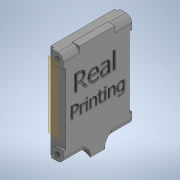
# Autodesk Inventor part: Partcooling_Brace
Saved by Autodesk Inventor 2022 (Build 260153000, 153)
## iProperties
Created: 2021-11-28
Part Number: Partcooling_Brace
Material: Polycarbonate, Clear
Document SubType Name: Modeling
Designer: alexr
Density: 1.2 g/cm^3
Appearance: Polycarbonate - Clear
Mass: 4.68895 g
Surface Area: 35.8129 cm^2
Volume: 3.90746 cm^3
Author: alexr
Autodesk Inventor part; units mm, degrees
ref_plane "YZ Plane" through (0, 0, 0) normal (1, 0, 0) x (0, 1, 0)
ref_plane "XZ Plane" through (0, 0, 0) normal (0, 1, 0) x (-1, 0, 0)
ref_plane "XY Plane" through (0, 0, 0) normal (0, 0, 1) x (1, 0, 0)
sketch "Sketch1" plane through (0, 0, 0) normal (1, 0, 0) x (0, 1, 0)
  line L0 (-12.75, -13.5) -> (12.75, -13.5)
  line L1 (12.75, -13.5) -> (12.75, 13.5)
  line L2 (12.75, 13.5) -> (-12.75, 13.5)
  line L3 (-12.75, 13.5) -> (-12.75, -13.5)
  line L4 (-12.75, -13.5) -> (12.75, 13.5) construction
  line L5 (12.75, -13.5) -> (-12.75, 13.5) construction
  dimension "d0" = 25.5
  dimension "d1" = 27
  constraints: 12 end point, 2 parallel, 1 horizontal, 1 perpendicular
  measures "d0" distance of L2.end L1.end
  measures "d1" distance of L1.end L0.end
extrude "Extrusion1" add sketch "Sketch1" along normal blind 6.25
ref_plane "Work Plane1" through (0, -12.75, 14.5) normal (0, 0, 1) x (1, 0, 0)
sketch "Sketch2" plane through (0, -12.75, 14.5) normal (0, 0, 1) x (1, 0, 0)
  arc A0 (6.25, 27.5) -> (3.75, 30) centre (3.75, 27.5) ccw projected
  line L0 (6.25, 27.5) -> (6.25, 25) projected
  line L1 (3.7511, 25) -> (6.25, 25) projected
  arc A1 (1.25, 27.5011) -> (3.7511, 25) centre (3.75, 27.5) ccw projected
  line L2 (1.25, 30) -> (1.25, 27.5011) projected
  line L3 (1.25, 30) -> (3.75, 30) projected
  circle A2 centre (3.75, 27.5) radius 1 projected
  arc A3 (3.75, -10) -> (6.25, -7.5) centre (3.75, -7.5) ccw projected
  line L4 (3.75, -10) -> (1.25, -10) projected
  line L5 (1.25, -7.5011) -> (1.25, -10) projected
  arc A4 (3.7511, -5) -> (1.25, -7.5011) centre (3.75, -7.5) ccw projected
  line L6 (6.25, -5) -> (3.7511, -5) projected
  line L7 (6.25, -5) -> (6.25, -7.5) projected
  circle A5 centre (3.75, -7.5) radius 1 projected
  point P0 (0, 12.75)
extrude "Extrusion2" add sketch "Sketch2" against normal blind 14.5
sketch "Sketch3" plane through (0, 12.75, 13.5) normal (0, 1, 0) x (1, 0, 0)
  line L0 (-19.75, 12.3932) -> (-19.75, 3.5868) projected
  line L1 (0, 0) -> (6.25, 0) projected
  line L2 (2.25, 13.5) -> (6.25, 13.5) projected
  line L3 (0, 0) -> (2.3102, 0)
  line L4 (2.3102, 0) -> (2.3102, 13.5)
  line L5 (2.3102, 13.5) -> (0, 13.5)
  line L6 (0, 13.5) -> (0, 0)
  constraints: 8 end point, 2 parallel, 1 horizontal, 1 perpendicular, 1 point on line
extrude "Extrusion3" add sketch "Sketch3" along normal blind 4.5
sketch "Sketch4" plane through (0, 0, 0) normal (-1, 0, 0) x (0, 0, 1)
  point P0 (0, 0)
sketch "Sketch5" plane through (0, -12.75, 13.5) normal (0, 0, 1) x (1, 0, 0)
  line L0 (0, 0) -> (6.25, 0) projected
  line L1 (0, 0) -> (0, -10)
  line L2 (1.25, -10) -> (3.75, -10) projected
  line L3 (0, -10) -> (1.25, -10)
  line L4 (6.25, 0) -> (6.25, -5)
  arc A0 (3.7511, -5) -> (1.25, -7.5011) centre (3.75, -7.5) ccw projected
  line L5 (6.25, -5) -> (3.7511, -5) projected
  line L6 (1.25, -7.5011) -> (1.25, -10) projected
  line L7 (6.25, -5) -> (3.7511, -5) projected
  line L8 (6.25, -5) -> (6.25, -5)
  line L9 (6.25, -5) -> (6.25, -5) construction
  point P0 (0, 12.75)
  dimension "d20" = 135
  constraints: 10 end point, 2 perpendicular, 1 equal length, 1 horizontal, 1 point on line, 1 vertical
  measures "d20" angle of L9 L8
extrude "Extrusion4" add sketch "Sketch5" against normal blind 14.5
mirror "Mirror2" about plane through (0, 0, 0) normal (0, 0, 1) of "Extrusion2", "Extrusion3", "Extrusion4"
sketch "Sketch6" plane through (6.25, 0, 0) normal (1, 0, 0) x (0, 0, -1)
  line L0 (13.75, 13.75) -> (-13.75, 13.75)
  line L1 (-7.75, 23.55) -> (-7.75, 17.35) projected
  line L2 (-7.75, 17.35) -> (11.25, 17.35) projected
  line L3 (14.5, 13.75) -> (-14.5, 13.75) projected
  line L4 (-7.75, 17.35) -> (7.25, 17.35)
  line L5 (7.25, 17.35) -> (7.25, 13.75)
  line L6 (7.25, 13.75) -> (-7.75, 13.75)
  line L7 (-7.75, 13.75) -> (-7.75, 17.35)
  line L8 (11.25, 23.55) -> (11.25, 17.35) projected
  line L9 (14.5, 13.75) -> (-14.5, 13.75) projected
  line L10 (7.25, 17.35) -> (11.25, 17.35)
  line L11 (11.25, 17.35) -> (11.25, 13.75)
  line L12 (11.25, 13.75) -> (7.25, 13.75)
  line L13 (7.25, 13.75) -> (7.25, 17.35)
  line L14 (-7.75, 23.55) -> (11.25, 23.55) projected
  line L15 (11.25, 23.55) -> (11.25, 17.35) projected
  point P0 (0, 0)
  point P1 (-7.75, 13.75)
  point P2 (7.25, 17.35)
  constraints: 18 end point, 4 parallel, 2 horizontal, 2 perpendicular, 2 point on line
extrude "Extrusion5" add sketch "Sketch6" against normal blind 3 contours L0 L7 L2 L5
sketch "Sketch7" plane through (3.75, 17.25, -14.5) normal (0, 0, -1) x (-1, 0, 0)
  circle A0 centre (0, -2.5) radius 1 projected
  point P0 (3.75, -17.25)
extrude "Extrusion6" cut sketch "Sketch7" against normal blind 30
sketch "Sketch9" plane through (1.25, -22.75, 14.5) normal (0, -1, 0) x (1, 0, 0)
  line L0 (5, -15.25) -> (5, -27.5) projected
  line L1 (-7.5, -11.5) -> (5, -11.5)
  line L2 (5, -11.5) -> (5, -17.5)
  line L3 (5, -17.5) -> (-7.5, -17.5)
  line L4 (-7.5, -17.5) -> (-7.5, -11.5)
  line L5 (-7.5, -11.5) -> (5, -17.5) construction
  line L6 (5, -11.5) -> (-7.5, -17.5) construction
  line L7 (-1.25, -1) -> (-1.25, -28) projected
  point P0 (-1.25, -14.5)
  point P1 (-1.25, -11.5)
  point P2 (-1.25, -17.5)
  dimension "d31" = 6
  constraints: 12 end point, 2 midpoint, 2 parallel, 1 horizontal, 1 perpendicular, 1 point on line
  measures "d31" distance of L1.end L2.end
extrude "Extrusion8" add sketch "Sketch9" along normal mid plane 6 contours L0 L3 L7 L1 L2
chamfer "Chamfer1" distance 6 distance2 3 1 edges at (0, -25.75, 0) measured on face at (0.5, -25.75, 0)
fillet "Fillet1" radius 3 4 edges at (1.875, -22.75, -3) (5.5178, -22.0178, -3) (1.875, -22.75, 3) (5.5178, -22.0178, 3)
sketch "Sketch10" plane through (6.25, 0, 0) normal (1, 0, 0) x (0, 0, -1)
  line L0 (-11.8056, 8.5303) -> (11.8056, 8.5303) construction
  line L1 (11.8056, 8.5303) -> (11.8056, -8.5303) construction
  line L2 (11.8056, -8.5303) -> (-11.8056, -8.5303) construction
  line L3 (-11.8056, -8.5303) -> (-11.8056, 8.5303) construction
  line L4 (-4.2738, 1.1034) -> (-5.5011, 1.1034)
  line L5 (-5.5011, 1.1034) -> (-7.7482, 3.9324)
  line L6 (-7.7482, 3.9324) -> (-8.8314, 3.9324)
  line L7 (-8.8314, 3.9324) -> (-8.8314, 1.1034)
  line L8 (-8.8314, 1.1034) -> (-9.7763, 1.1034)
  line L9 (-9.7763, 1.1034) -> (-9.7763, 8.2134)
  line L10 (-9.7763, 8.2134) -> (-7.9441, 8.2134)
  spline S0 degree 2 poles (-7.9441, 8.2134) (-7.3333, 8.2134) (-6.5094, 8.0809) (-6.1349, 7.8389) knots 0 0 0 1 2 2 2
  spline S1 degree 2 poles (-6.1349, 7.8389) (-5.7604, 7.5969) (-5.3282, 6.8421) (-5.3282, 6.2832) knots 0 0 0 1 2 2 2
  spline S2 degree 2 poles (-5.3282, 6.2832) (-5.3282, 5.5054) (-6.1234, 4.451) (-6.8032, 4.1975) knots 0 0 0 1 2 2 2
  line L11 (-6.8032, 4.1975) -> (-4.2738, 1.1034)
  spline S3 degree 2 poles (-6.3135, 6.2083) (-6.3135, 6.5194) (-6.5324, 6.9977) (-6.7629, 7.1532) knots 0 0 0 1 2 2 2
  spline S4 degree 2 poles (-6.7629, 7.1532) (-6.9646, 7.2858) (-7.5004, 7.3952) (-7.8922, 7.3952) knots 0 0 0 1 2 2 2
  line L12 (-7.8922, 7.3952) -> (-8.8314, 7.3952)
  line L13 (-8.8314, 7.3952) -> (-8.8314, 4.7218)
  line L14 (-8.8314, 4.7218) -> (-8.0017, 4.7218)
  spline S5 degree 2 poles (-8.0017, 4.7218) (-7.5926, 4.7218) (-6.9415, 4.8658) (-6.7168, 5.0905) knots 0 0 0 1 2 2 2
  spline S6 degree 2 poles (-6.7168, 5.0905) (-6.5094, 5.2864) (-6.3135, 5.8396) (-6.3135, 6.2083) knots 0 0 0 1 2 2 2
  spline S7 degree 2 poles (-1.4621, 0.9824) (-2.7412, 0.9824) (-4.1471, 2.4171) (-4.1471, 3.7423) knots 0 0 0 1 2 2 2
  spline S8 degree 2 poles (-4.1471, 3.7423) (-4.1471, 5.0444) (-2.7815, 6.5886) (-1.6811, 6.5886) knots 0 0 0 1 2 2 2
  spline S9 degree 2 poles (-1.6811, 6.5886) (-1.1855, 6.5886) (-0.4192, 6.3005) (-0.1369, 5.9951) knots 0 0 0 1 2 2 2
  spline S10 degree 2 poles (-0.1369, 5.9951) (0.1512, 5.6898) (0.4566, 4.8082) (0.4566, 4.1687) knots 0 0 0 1 2 2 2
  line L15 (0.4566, 4.1687) -> (0.4566, 3.6789)
  line L16 (0.4566, 3.6789) -> (-3.2367, 3.6789)
  spline S11 degree 2 poles (-3.2367, 3.6789) (-3.2367, 2.7513) (-2.3033, 1.766) (-1.4736, 1.766) knots 0 0 0 1 2 2 2
  spline S12 degree 2 poles (-1.4736, 1.766) (-1.1798, 1.766) (-0.6094, 1.8985) (-0.3789, 2.0022) knots 0 0 0 1 2 2 2
  spline S13 degree 2 poles (-0.3789, 2.0022) (-0.1369, 2.1175) (0.1973, 2.3191) (0.3068, 2.4113) knots 0 0 0 1 2 2 2
  line L17 (0.3068, 2.4113) -> (0.3586, 2.4113)
  line L18 (0.3586, 2.4113) -> (0.3586, 1.4318)
  spline S14 degree 2 poles (0.3586, 1.4318) (0.203, 1.3684) (-0.2694, 1.1841) (-0.4538, 1.1322) knots 0 0 0 1 2 2 2
  spline S15 degree 2 poles (-0.4538, 1.1322) (-0.7131, 1.0573) (-1.1394, 0.9824) (-1.4621, 0.9824) knots 0 0 0 1 2 2 2
  spline S16 degree 2 poles (-0.4192, 4.3645) (-0.4308, 4.7275) (-0.5806, 5.2576) (-0.7246, 5.4362) knots 0 0 0 1 2 2 2
  spline S17 degree 2 poles (-0.7246, 5.4362) (-0.8802, 5.6379) (-1.3699, 5.8511) (-1.7329, 5.8511) knots 0 0 0 1 2 2 2
  spline S18 degree 2 poles (-1.7329, 5.8511) (-2.0901, 5.8511) (-2.5914, 5.6379) (-2.7988, 5.4305) knots 0 0 0 1 2 2 2
  spline S19 degree 2 poles (-2.7988, 5.4305) (-3.0005, 5.2173) (-3.2079, 4.7045) (-3.2367, 4.3645) knots 0 0 0 1 2 2 2
  line L19 (-3.2367, 4.3645) -> (-0.4192, 4.3645)
  spline S20 degree 2 poles (4.34, 1.6681) (4.2305, 1.5874) (3.8618, 1.2993) (3.6889, 1.2129) knots 0 0 0 1 2 2 2
  spline S21 degree 2 poles (3.6889, 1.2129) (3.4527, 1.0861) (3.009, 0.9536) (2.6057, 0.9536) knots 0 0 0 1 2 2 2
  spline S22 degree 2 poles (2.6057, 0.9536) (2.2773, 0.9536) (1.6838, 1.2013) (1.4591, 1.4261) knots 0 0 0 1 2 2 2
  spline S23 degree 2 poles (1.4591, 1.4261) (1.2459, 1.645) (0.9866, 2.2903) (0.9866, 2.6475) knots 0 0 0 1 2 2 2
  spline S24 degree 2 poles (0.9866, 2.6475) (0.9866, 3.2007) (1.4533, 3.9843) (1.9604, 4.209) knots 0 0 0 1 2 2 2
  spline S25 degree 2 poles (1.9604, 4.209) (2.4098, 4.4164) (3.6313, 4.572) (4.34, 4.6123) knots 0 0 0 1 2 2 2
  line L20 (4.34, 4.6123) -> (4.34, 4.7852)
  spline S26 degree 2 poles (4.34, 4.7852) (4.34, 5.0963) (4.1498, 5.4823) (3.977, 5.5918) knots 0 0 0 1 2 2 2
  spline S27 degree 2 poles (3.977, 5.5918) (3.8041, 5.7013) (3.3086, 5.7704) (3.0436, 5.7704) knots 0 0 0 1 2 2 2
  spline S28 degree 2 poles (3.0436, 5.7704) (2.7324, 5.7704) (1.8912, 5.586) (1.4706, 5.4074) knots 0 0 0 1 2 2 2
  line L21 (1.4706, 5.4074) -> (1.4188, 5.4074)
  line L22 (1.4188, 5.4074) -> (1.4188, 6.3235)
  spline S29 degree 2 poles (1.4188, 6.3235) (1.6665, 6.3927) (2.5942, 6.5655) (3.0493, 6.5655) knots 0 0 0 1 2 2 2
  spline S30 degree 2 poles (3.0493, 6.5655) (3.6025, 6.5655) (4.3573, 6.3927) (4.6569, 6.168) knots 0 0 0 1 2 2 2
  spline S31 degree 2 poles (4.6569, 6.168) (4.9507, 5.949) (5.2388, 5.2519) (5.2388, 4.7506) knots 0 0 0 1 2 2 2
  line L23 (5.2388, 4.7506) -> (5.2388, 1.1034)
  line L24 (5.2388, 1.1034) -> (4.34, 1.1034)
  line L25 (4.34, 1.1034) -> (4.34, 1.6681)
  line L26 (4.34, 2.4171) -> (4.34, 3.8978)
  spline S32 degree 2 poles (4.34, 3.8978) (4.0173, 3.869) (3.0436, 3.7711) (2.7382, 3.6789) knots 0 0 0 1 2 2 2
  spline S33 degree 2 poles (2.7382, 3.6789) (2.381, 3.5694) (1.9143, 3.1142) (1.9143, 2.7109) knots 0 0 0 1 2 2 2
  spline S34 degree 2 poles (1.9143, 2.7109) (1.9143, 2.25) (2.4328, 1.7833) (2.9283, 1.7833) knots 0 0 0 1 2 2 2
  spline S35 degree 2 poles (2.9283, 1.7833) (3.349, 1.7833) (4.0404, 2.1463) (4.34, 2.4171) knots 0 0 0 1 2 2 2
  line L27 (7.4168, 1.1034) -> (6.5179, 1.1034)
  line L28 (6.5179, 1.1034) -> (6.5179, 8.5303)
  line L29 (6.5179, 8.5303) -> (7.4168, 8.5303)
  line L30 (7.4168, 8.5303) -> (7.4168, 1.1034)
  spline S36 degree 2 poles (-8.08, -4.4955) (-8.08, -4.8248) (-8.3147, -5.4176) (-8.5246, -5.6234) knots 0 0 0 1 2 2 2
  spline S37 degree 2 poles (-8.5246, -5.6234) (-8.7881, -5.8828) (-9.5003, -6.1504) (-10.0437, -6.1504) knots 0 0 0 1 2 2 2
  line L31 (-10.0437, -6.1504) -> (-10.6159, -6.1504)
  line L32 (-10.6159, -6.1504) -> (-10.6159, -8.0441)
  line L33 (-10.6159, -8.0441) -> (-11.2911, -8.0441)
  line L34 (-11.2911, -8.0441) -> (-11.2911, -2.9641)
  line L35 (-11.2911, -2.9641) -> (-10.0149, -2.9641)
  spline S38 degree 2 poles (-10.0149, -2.9641) (-9.562, -2.9641) (-8.9281, -3.1123) (-8.6852, -3.281) knots 0 0 0 1 2 2 2
  spline S39 degree 2 poles (-8.6852, -3.281) (-8.4011, -3.4745) (-8.08, -4.0714) (-8.08, -4.4955) knots 0 0 0 1 2 2 2
  spline S40 degree 2 poles (-8.784, -4.516) (-8.784, -4.2526) (-8.9651, -3.8656) (-9.1504, -3.7421) knots 0 0 0 1 2 2 2
  spline S41 degree 2 poles (-9.1504, -3.7421) (-9.3109, -3.6351) (-9.7391, -3.5486) (-10.056, -3.5486) knots 0 0 0 1 2 2 2
  line L36 (-10.056, -3.5486) -> (-10.6159, -3.5486)
  line L37 (-10.6159, -3.5486) -> (-10.6159, -5.574)
  line L38 (-10.6159, -5.574) -> (-10.1548, -5.574)
  spline S42 degree 2 poles (-10.1548, -5.574) (-9.7432, -5.574) (-9.2368, -5.4423) (-9.0722, -5.2694) knots 0 0 0 1 2 2 2
  spline S43 degree 2 poles (-9.0722, -5.2694) (-8.9198, -5.1171) (-8.784, -4.7589) (-8.784, -4.516) knots 0 0 0 1 2 2 2
  line L39 (-5.4659, -4.9195) -> (-5.4989, -4.9195)
  spline S44 degree 2 poles (-5.4989, -4.9195) (-5.573, -4.8989) (-5.7335, -4.8907) (-5.8447, -4.8907) knots 0 0 0 1 2 2 2
  spline S45 degree 2 poles (-5.8447, -4.8907) (-6.104, -4.8907) (-6.6145, -5.1171) (-6.845, -5.3394) knots 0 0 0 1 2 2 2
  line L40 (-6.845, -5.3394) -> (-6.845, -8.0441)
  line L41 (-6.845, -8.0441) -> (-7.4872, -8.0441)
  line L42 (-7.4872, -8.0441) -> (-7.4872, -4.232)
  line L43 (-7.4872, -4.232) -> (-6.845, -4.232)
  line L44 (-6.845, -4.232) -> (-6.845, -4.8001)
  spline S46 degree 2 poles (-6.845, -4.8001) (-6.4951, -4.4872) (-5.9723, -4.232) (-5.7253, -4.232) knots 0 0 0 1 2 2 2
  spline S47 degree 2 poles (-5.7253, -4.232) (-5.6265, -4.232) (-5.5277, -4.2402) (-5.4659, -4.2526) knots 0 0 0 1 2 2 2
  line L45 (-5.4659, -4.2526) -> (-5.4659, -4.9195)
  line L46 (-4.3133, -8.0441) -> (-4.9555, -8.0441)
  line L47 (-4.9555, -8.0441) -> (-4.9555, -4.232)
  line L48 (-4.9555, -4.232) -> (-4.3133, -4.232)
  line L49 (-4.3133, -4.232) -> (-4.3133, -8.0441)
  line L50 (-4.268, -3.598) -> (-4.9966, -3.598)
  line L51 (-4.9966, -3.598) -> (-4.9966, -2.9311)
  line L52 (-4.9966, -2.9311) -> (-4.268, -2.9311)
  line L53 (-4.268, -2.9311) -> (-4.268, -3.598)
  line L54 (-0.3777, -8.0441) -> (-1.0199, -8.0441)
  line L55 (-1.0199, -8.0441) -> (-1.0199, -5.8704)
  spline S48 degree 2 poles (-1.0199, -5.8704) (-1.0199, -5.607) (-1.0693, -5.1541) (-1.1434, -5.0183) knots 0 0 0 1 2 2 2
  spline S49 degree 2 poles (-1.1434, -5.0183) (-1.2216, -4.8742) (-1.5016, -4.7342) (-1.7403, -4.7342) knots 0 0 0 1 2 2 2
  spline S50 degree 2 poles (-1.7403, -4.7342) (-1.9791, -4.7342) (-2.4854, -4.9895) (-2.7283, -5.1953) knots 0 0 0 1 2 2 2
  line L56 (-2.7283, -5.1953) -> (-2.7283, -8.0441)
  line L57 (-2.7283, -8.0441) -> (-3.3705, -8.0441)
  line L58 (-3.3705, -8.0441) -> (-3.3705, -4.232)
  line L59 (-3.3705, -4.232) -> (-2.7283, -4.232)
  line L60 (-2.7283, -4.232) -> (-2.7283, -4.656)
  spline S51 degree 2 poles (-2.7283, -4.656) (-2.4402, -4.3967) (-1.8844, -4.125) (-1.5715, -4.125) knots 0 0 0 1 2 2 2
  spline S52 degree 2 poles (-1.5715, -4.125) (-1.0117, -4.125) (-0.3777, -4.866) (-0.3777, -5.5699) knots 0 0 0 1 2 2 2
  line L61 (-0.3777, -5.5699) -> (-0.3777, -8.0441)
  spline S53 degree 2 poles (1.6765, -8.1182) (1.1537, -8.1182) (0.565, -7.5212) (0.565, -6.8749) knots 0 0 0 1 2 2 2
  line L62 (0.565, -6.8749) -> (0.565, -4.763)
  line L63 (0.565, -4.763) -> (0.1328, -4.763)
  line L64 (0.1328, -4.763) -> (0.1328, -4.232)
  line L65 (0.1328, -4.232) -> (0.565, -4.232)
  line L66 (0.565, -4.232) -> (0.565, -3.137)
  line L67 (0.565, -3.137) -> (1.2072, -3.137)
  line L68 (1.2072, -3.137) -> (1.2072, -4.232)
  line L69 (1.2072, -4.232) -> (2.3887, -4.232)
  line L70 (2.3887, -4.232) -> (2.3887, -4.763)
  line L71 (2.3887, -4.763) -> (1.2072, -4.763)
  line L72 (1.2072, -4.763) -> (1.2072, -6.5785)
  spline S54 degree 2 poles (1.2072, -6.5785) (1.2072, -6.8667) (1.2278, -7.1837) (1.2978, -7.3195) knots 0 0 0 1 2 2 2
  spline S55 degree 2 poles (1.2978, -7.3195) (1.3554, -7.4389) (1.6148, -7.5583) (1.8371, -7.5583) knots 0 0 0 1 2 2 2
  spline S56 degree 2 poles (1.8371, -7.5583) (1.9935, -7.5583) (2.2858, -7.4636) (2.3517, -7.4348) knots 0 0 0 1 2 2 2
  line L73 (2.3517, -7.4348) -> (2.3887, -7.4348)
  line L74 (2.3887, -7.4348) -> (2.3887, -8.0111)
  spline S57 degree 2 poles (2.3887, -8.0111) (2.2076, -8.0605) (1.8371, -8.1182) (1.6765, -8.1182) knots 0 0 0 1 2 2 2
  line L75 (3.5167, -8.0441) -> (2.8745, -8.0441)
  line L76 (2.8745, -8.0441) -> (2.8745, -4.232)
  line L77 (2.8745, -4.232) -> (3.5167, -4.232)
  line L78 (3.5167, -4.232) -> (3.5167, -8.0441)
  line L79 (3.562, -3.598) -> (2.8333, -3.598)
  line L80 (2.8333, -3.598) -> (2.8333, -2.9311)
  line L81 (2.8333, -2.9311) -> (3.562, -2.9311)
  line L82 (3.562, -2.9311) -> (3.562, -3.598)
  line L83 (7.4523, -8.0441) -> (6.81, -8.0441)
  line L84 (6.81, -8.0441) -> (6.81, -5.8704)
  spline S58 degree 2 poles (6.81, -5.8704) (6.81, -5.607) (6.7606, -5.1541) (6.6865, -5.0183) knots 0 0 0 1 2 2 2
  spline S59 degree 2 poles (6.6865, -5.0183) (6.6083, -4.8742) (6.3284, -4.7342) (6.0896, -4.7342) knots 0 0 0 1 2 2 2
  spline S60 degree 2 poles (6.0896, -4.7342) (5.8509, -4.7342) (5.3445, -4.9895) (5.1016, -5.1953) knots 0 0 0 1 2 2 2
  line L85 (5.1016, -5.1953) -> (5.1016, -8.0441)
  line L86 (5.1016, -8.0441) -> (4.4594, -8.0441)
  line L87 (4.4594, -8.0441) -> (4.4594, -4.232)
  line L88 (4.4594, -4.232) -> (5.1016, -4.232)
  line L89 (5.1016, -4.232) -> (5.1016, -4.656)
  spline S61 degree 2 poles (5.1016, -4.656) (5.3898, -4.3967) (5.9455, -4.125) (6.2584, -4.125) knots 0 0 0 1 2 2 2
  spline S62 degree 2 poles (6.2584, -4.125) (6.8183, -4.125) (7.4523, -4.866) (7.4523, -5.5699) knots 0 0 0 1 2 2 2
  line L90 (7.4523, -5.5699) -> (7.4523, -8.0441)
  spline S63 degree 2 poles (8.4897, -8.6533) (8.5555, -8.6821) (8.8066, -8.7727) (8.9672, -8.8098) knots 0 0 0 1 2 2 2
  spline S64 degree 2 poles (8.9672, -8.8098) (9.1442, -8.855) (9.4447, -8.9086) (9.6218, -8.9086) knots 0 0 0 1 2 2 2
  spline S65 degree 2 poles (9.6218, -8.9086) (9.9182, -8.9086) (10.3298, -8.7521) (10.4451, -8.6122) knots 0 0 0 1 2 2 2
  spline S66 degree 2 poles (10.4451, -8.6122) (10.5562, -8.4722) (10.6427, -8.1058) (10.6427, -7.8712) knots 0 0 0 1 2 2 2
  line L91 (10.6427, -7.8712) -> (10.6427, -7.5377)
  spline S67 degree 2 poles (10.6427, -7.5377) (10.3833, -7.7641) (9.8852, -7.9782) (9.5106, -7.9782) knots 0 0 0 1 2 2 2
  spline S68 degree 2 poles (9.5106, -7.9782) (8.8602, -7.9782) (8.0903, -7.0108) (8.0903, -6.101) knots 0 0 0 1 2 2 2
  spline S69 degree 2 poles (8.0903, -6.101) (8.0903, -5.6276) (8.3579, -4.8948) (8.5802, -4.6354) knots 0 0 0 1 2 2 2
  spline S70 degree 2 poles (8.5802, -4.6354) (8.7943, -4.3925) (9.383, -4.125) (9.6959, -4.125) knots 0 0 0 1 2 2 2
  spline S71 degree 2 poles (9.6959, -4.125) (9.9923, -4.125) (10.4245, -4.2649) (10.6427, -4.3925) knots 0 0 0 1 2 2 2
  line L92 (10.6427, -4.3925) -> (10.6797, -4.232)
  line L93 (10.6797, -4.232) -> (11.2849, -4.232)
  line L94 (11.2849, -4.232) -> (11.2849, -7.6077)
  spline S72 degree 2 poles (11.2849, -7.6077) (11.2849, -8.5792) (10.441, -9.4849) (9.5724, -9.4849) knots 0 0 0 1 2 2 2
  spline S73 degree 2 poles (9.5724, -9.4849) (9.2924, -9.4849) (8.7078, -9.3943) (8.4567, -9.3202) knots 0 0 0 1 2 2 2
  line L95 (8.4567, -9.3202) -> (8.4567, -8.6533)
  line L96 (8.4567, -8.6533) -> (8.4897, -8.6533)
  line L97 (10.6427, -7.0108) -> (10.6427, -4.9154)
  spline S74 degree 2 poles (10.6427, -4.9154) (10.4039, -4.8001) (10.0005, -4.7013) (9.7988, -4.7013) knots 0 0 0 1 2 2 2
  spline S75 degree 2 poles (9.7988, -4.7013) (9.313, -4.7013) (8.7531, -5.4176) (8.7531, -6.0886) knots 0 0 0 1 2 2 2
  spline S76 degree 2 poles (8.7531, -6.0886) (8.7531, -6.7226) (9.1771, -7.3854) (9.6547, -7.3854) knots 0 0 0 1 2 2 2
  spline S77 degree 2 poles (9.6547, -7.3854) (9.9058, -7.3854) (10.4327, -7.1878) (10.6427, -7.0108) knots 0 0 0 1 2 2 2
  point P0 (0, 0)
  dimension "d42" = 17.0606
  dimension "d43" = 23.6113
  dimension "d44" = 8.5303
  dimension "d45" = 11.8056
  constraints: 2 other
  measures "d42" distance of L2.end L0.start
  measures "d43" distance of L1.end L2.end
  measures "d44" distance from line of L0 point (0, 0)
  measures "d45" distance from line of point (0, 0) L3
extrude "Extrusion9" cut sketch "Sketch10" against normal blind 1
equation "\"d44\" = 0.5 * d42"
equation "\"d45\" = 0.5 * d43"
body "Solid1"
